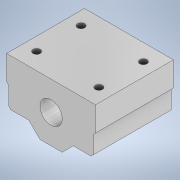
# Autodesk Inventor part: LinearBearing_SC10UU
Saved by Autodesk Inventor 2022 (Build 260153000, 153)
## iProperties
Created: 2021-06-15
Part Number: LinearBearing_SC10UU
Material: Generic
Document SubType Name: Modeling
Designer: burgessb
Density: 1 g/cm^3
Appearance: Aluminum - Dark
Author: burgessb
Autodesk Inventor part; units mm, degrees
ref_plane "YZ Plane" through (0, 0, 0) normal (1, 0, 0) x (0, 1, 0)
ref_plane "XZ Plane" through (0, 0, 0) normal (0, 1, 0) x (-1, 0, 0)
ref_plane "XY Plane" through (0, 0, 0) normal (0, 0, 1) x (1, 0, 0)
sketch "Sketch1" plane through (0, 0, 0) normal (0, 0, 1) x (1, 0, 0)
  circle A0 centre (0, 0) radius 5
  circle A1 centre (0, 0) radius 8
  line L0 (0, 13) -> (20, 13)
  line L1 (20, 13) -> (20, 2)
  line L2 (10, -8) -> (5, -13)
  line L3 (5, -13) -> (0, -13)
  line L4 (10, -8) -> (19, -8)
  line L5 (19, -8) -> (19, 1)
  line L6 (19, 1) -> (20, 2)
  line L7 (0, 19.5854) -> (0, -21.9543) construction
  line L8 (0, 13) -> (-20, 13)
  line L9 (-20, 13) -> (-20, 2)
  line L10 (-10, -8) -> (-5, -13)
  line L11 (-5, -13) -> (0, -13)
  line L12 (-10, -8) -> (-19, -8)
  line L13 (-19, -8) -> (-19, 1)
  line L14 (-19, 1) -> (-20, 2)
  dimension "d0" = 10
  dimension "d8" = 16
  dimension "d27" = 20
  dimension "d28" = 0
  dimension "d29" = 0
  dimension "d30" = 135
  dimension "d31" = 26
  dimension "d32" = 13
  dimension "d34" = 21
  dimension "d35" = 135
  dimension "d36" = 12
  dimension "d37" = 19
  dimension "d38" = 5
  dimension "d39" = 0
  constraints: 30 end point, 6 symmetric about line, 2 centre point, 2 coincident, 2 horizontal, 2 perpendicular, 1 parallel, 1 vertical
  measures "d0" diameter of A0
  measures "d8" diameter of A1
  measures "d27" distance of L0.start L0.end
  measures "d28" horizontal distance of point (0, 0) L0.start
  measures "d29" horizontal distance of point (0, 0) L3.end
  measures "d30" angle of L3 L2
  measures "d31" distance between parallel lines of L3 L0
  measures "d32" distance from line of point (0, 0) L0
  measures "d34" distance from line of L0 L2.start
  measures "d35" angle of L5 L6
  measures "d36" distance from line of L0 L5.end
  measures "d37" distance from line of point (0, 0) L5
  measures "d38" distance of L2.end L3.end
  measures "d39" distance from line of point (0, 0) L7
extrude "Extrusion1" add sketch "Sketch1" along normal blind 35 contours A1 | L0 L1 L6 L5 L4 L2 L3 L11 L10 L12 L13 L14 L9 L8
chamfer "Chamfer1" distance 1 angle 45 2 edges at (19, -8, 17.5) (-19, -8, 17.5)
sketch "Sketch3" plane through (-20, 13, 0) normal (0, 1, 0) x (1, 0, 0)
  line L0 (40, 0) -> (0, 0) projected
  line L1 (0, 0) -> (0, -35) projected
  line L2 (40, -35) -> (0, -35) projected
  line L3 (40, 0) -> (40, -35) projected
  point P0 (20, 0)
  point P1 (6, -27.5)
  point P2 (6, -7.5)
  point P3 (34, -27.5)
  point P4 (34, -7.5)
  dimension "d45" = 20
  dimension "d48" = 28
  dimension "d51" = 6
  dimension "d52" = 7.5
  constraints: 1 horizontal, 1 vertical, 3 other
  measures "d45" distance of point (6, -27.5) point (6, -7.5)
  measures "d48" distance of point (6, -27.5) point (34, -27.5)
  measures "d51" distance from line of L1 point (6, -27.5)
  measures "d52" distance from line of L2 point (34, -27.5)
hole "Hole2" at (-14, 13, 27.5) at (-14, 13, 7.5) at (14, 13, 27.5) at (14, 13, 7.5) direction (0, -1, 0) diameter 3.242 end through all thread size "M4x0.7" class "6H" standard "ANSI Metric M Profile"
body "Solid1"
